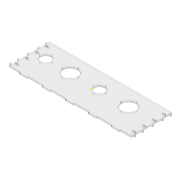
# Autodesk Inventor part: plano 1
Saved by Autodesk Inventor 2016 (Build 200138000, 138)
## iProperties
Created: 2017-08-31
Part Number: plano 1
Material: Vidrio
Document SubType Name: Modeling
Designer: Alumno
Density: 2.18 g/cm^3
Appearance: Claro
Author: Alumno
Autodesk Inventor part; units mm, degrees
ref_plane "YZ Plane" through (0, 0, 0) normal (1, 0, 0) x (0, 1, 0)
ref_plane "XZ Plane" through (0, 0, 0) normal (0, 1, 0) x (-1, 0, 0)
ref_plane "XY Plane" through (0, 0, 0) normal (0, 0, 1) x (1, 0, 0)
sketch "Boceto1" plane through (0, 0, 0) normal (0, 0, 1) x (1, 0, 0)
  line L0 (225, -75) -> (-225, -75)
  line L1 (-225, -75) -> (-225, 75)
  line L2 (-225, 75) -> (225, 75)
  line L3 (225, 75) -> (225, -75)
  line L4 (225, -75) -> (-225, 75) construction
  line L5 (-225, -75) -> (225, 75) construction
  point P0 (0, 0)
  dimension "d0" = 450
  dimension "d1" = 150
  constraints: 12 end point, 2 midpoint, 2 parallel, 1 horizontal, 1 perpendicular
  measures "d0" distance of L1.end L2.end
  measures "d1" distance of L0.end L1.end
extrude "Extrusión1" add sketch "Boceto1" along normal blind 6
sketch "Boceto2" plane through (0, 0, 6) normal (0, 0, 1) x (1, 0, 0)
  line L0 (-225, -75) -> (225, -75) projected
  line L1 (225, -75) -> (225, 75) projected
  line L2 (225, 75) -> (-225, 75) projected
  line L3 (-225, 75) -> (-225, -75) projected
  line L4 (-210, 57) -> (-210, 53.65)
  line L5 (-225, 53.65) -> (-225, 57)
  line L6 (-216, 52.35) -> (-218.8, 52.35)
  line L7 (-218.8, 58.3) -> (-216, 58.3)
  line L8 (-216, 58.3) -> (-216, 57)
  line L9 (-216, 53.65) -> (-216, 52.35)
  line L10 (-218.8, 52.35) -> (-218.8, 53.65)
  line L11 (-218.8, 57) -> (-218.8, 58.3)
  line L12 (-225, 57) -> (-218.8, 57)
  line L13 (-216, 57) -> (-210, 57)
  line L14 (-210, 53.65) -> (-216, 53.65)
  line L15 (-218.8, 53.65) -> (-225, 53.65)
  line L16 (-210, -53.65) -> (-210, -57)
  line L17 (-225, -57) -> (-225, -53.65)
  line L18 (-216, -58.3) -> (-218.8, -58.3)
  line L19 (-218.8, -52.35) -> (-216, -52.35)
  line L20 (-216, -52.35) -> (-216, -53.65)
  line L21 (-216, -57) -> (-216, -58.3)
  line L22 (-218.8, -58.3) -> (-218.8, -57)
  line L23 (-218.8, -53.65) -> (-218.8, -52.35)
  line L24 (-225, -53.65) -> (-218.8, -53.65)
  line L25 (-216, -53.65) -> (-210, -53.65)
  line L26 (-210, -57) -> (-216, -57)
  line L27 (-218.8, -57) -> (-225, -57)
  line L28 (-210, -16.7667) -> (-210, -20.1167)
  line L29 (-225, -20.1167) -> (-225, -16.7667)
  line L30 (-216, -15.4667) -> (-218.8, -15.4667)
  line L31 (-218.8, -21.4167) -> (-216, -21.4167)
  line L32 (-216, -16.7667) -> (-216, -15.4667)
  line L33 (-218.8, -15.4667) -> (-218.8, -16.7667)
  line L34 (-218.8, -20.1167) -> (-218.8, -21.4167)
  line L35 (-225, -16.7667) -> (-218.8, -16.7667)
  line L36 (-216, -16.7667) -> (-210, -16.7667)
  line L37 (-210, -20.1167) -> (-216, -20.1167)
  line L38 (-218.8, -20.1167) -> (-225, -20.1167)
  line L39 (-210, 20.1167) -> (-210, 16.7667)
  line L40 (-225, 16.7667) -> (-225, 20.1167)
  line L41 (-216, 15.4667) -> (-218.8, 15.4667)
  line L42 (-218.8, 21.4167) -> (-216, 21.4167)
  line L43 (-216, 21.4167) -> (-216, 20.1167)
  line L44 (-216, 16.7667) -> (-216, 15.4667)
  line L45 (-218.8, 15.4667) -> (-218.8, 16.7667)
  line L46 (-218.8, 20.1167) -> (-218.8, 21.4167)
  line L47 (-225, 20.1167) -> (-218.8, 20.1167)
  line L48 (-216, 20.1167) -> (-210, 20.1167)
  line L49 (-210, 16.7667) -> (-216, 16.7667)
  line L50 (-218.8, 16.7667) -> (-225, 16.7667)
  line L51 (-216, -21.4167) -> (-216, -20.1167)
  line L52 (-225, 75) -> (-225, -75) projected
  point P0 (0, 0)
  point P1 (-216.3708, 45.3131)
  point P2 (-225, 57)
  dimension "d5" = 3.35
  dimension "d6" = 2.8
  dimension "d8" = 6
  dimension "d9" = 6
  dimension "d11" = 3.35
  dimension "d12" = 18
  dimension "d46" = 15
  dimension "d47" = 3.35
  dimension "d48" = 2.8
  dimension "d49" = 2.8
  dimension "d52" = 3.35
  dimension "d53" = 15
  dimension "d54" = 3.35
  dimension "d60" = 15
  dimension "d61" = 3.35
  dimension "d62" = 2.8
  dimension "d63" = 2.8
  dimension "d66" = 3.35
  dimension "d67" = 18
  dimension "d71" = 107.3
  dimension "d72" = 33.5333
  dimension "d73" = 33.5333
  dimension "d74" = 5.95
  dimension "d76" = 5.95
  dimension "d77" = 1.3
  dimension "d78" = 5.95
  dimension "d79" = 1.3
  dimension "d80" = 1.3
  dimension "d81" = 1.3
  dimension "d137" = 3.35
  dimension "d138" = 6.2
  dimension "d139" = 2.8
  dimension "d140" = 15
  dimension "d141" = 6.2
  dimension "d142" = 6.2
  dimension "d143" = 6.2
  dimension "d144" = 6.2
  dimension "d145" = 2.8
  dimension "d146" = 2.8
  dimension "d147" = 6.2
  dimension "d148" = 6.2
  constraints: 96 end point, 38 parallel, 16 perpendicular, 12 horizontal, 1 coincident, 1 point on line, 1 vertical
  measures "d5" distance of L4.start L4.end
  measures "d6" distance of L6.start L6.end
  measures "d8" distance between parallel lines of L8 L4
  measures "d9" distance between parallel lines of L9 L4
  measures "d11" distance between parallel lines of L15 L12
  measures "d12" distance between parallel lines of L2 L12
  measures "d46" distance of L16.end L27.end
  measures "d47" distance of L16.start L16.end
  measures "d48" distance of L21.end L22.start
  measures "d49" distance of L23.end L20.start
  measures "d52" distance between parallel lines of L27 L24
  measures "d53" distance of L28.end L38.end
  measures "d54" distance of L28.start L28.end
  measures "d60" distance of L39.end L50.end
  measures "d61" distance of L39.start L39.end
  measures "d62" distance of L44.end L45.start
  measures "d63" distance of L46.end L43.start
  measures "d66" distance between parallel lines of L50 L47
  measures "d67" distance between parallel lines of L0 L27
  measures "d71" distance between parallel lines of L24 L15
  measures "d72" distance between parallel lines of L47 L15
  measures "d73" distance between parallel lines of L35 L50
  measures "d74" distance between parallel lines of L18 L19
  measures "d76" distance between parallel lines of L6 L7
  measures "d77" distance between parallel lines of L48 L42
  measures "d78" distance between parallel lines of L41 L42
  measures "d79" distance between parallel lines of L35 L30
  measures "d80" distance between parallel lines of L31 L38
  measures "d81" distance between parallel lines of L24 L19
  measures "d137" distance between parallel lines of L14 L13
  measures "d138" distance of L5.end L11.start
  measures "d139" distance of L7.start L7.end
  measures "d140" distance between parallel lines of L4 L52
  measures "d141" distance of L47.start L46.start
  measures "d142" distance of L45.end L50.end
  measures "d143" distance of L35.start L33.end
  measures "d144" distance of L34.start L38.end
  measures "d145" distance of L32.end L33.start
  measures "d146" distance of L34.end L31.end
  measures "d147" distance of L24.start L23.start
  measures "d148" distance of L22.end L27.end
extrude "Extrusión2" cut sketch "Boceto2" against normal blind 6 contours L3 L24 L23 L19 L20 L25 L16 L26 L21 L18 L22 L27 | L12 L11 L7 L8 L13 L4 L14 L9 L6 L10 L15 L3 | L3 L47 L46 L42 L43 L48 L39 L49 L44 L41 L45 L50
extrude "Extrusión3" cut sketch "Boceto2" against normal blind 6 contours L3 L35 L33 L30 L32 L36 L28 L37 L51 L31 L34 L38
mirror "Simetría1" about plane through (0, 0, 0) normal (1, 0, 0) of "Extrusión3", "Extrusión2"
sketch "Boceto3" plane through (0, 0, 6) normal (0, 0, 1) x (1, 0, 0)
  line L0 (-225, -75) -> (225, -75) projected
  line L1 (-225, 75) -> (-225, -75) projected
  circle A0 centre (-180, 15) radius 19
  circle A1 centre (-90, 15) radius 21.5
  circle A2 centre (18, 15) radius 19
  circle A3 centre (126, 15) radius 21.5
  point P0 (-225, 53.65)
  point P1 (-225, 20.1167)
  dimension "d97" = 90
  dimension "d98" = 45
  dimension "d99" = 90
  dimension "d100" = 108
  dimension "d101" = 108
  dimension "d102" = 38
  dimension "d105" = 43
  dimension "d108" = 38
  dimension "d109" = 43
  constraints: 4 centre point, 4 coincident
  measures "d97" distance from line of L0 point (-180, 15)
  measures "d98" distance from line of L1 point (-180, 15)
  measures "d99" distance of point (-90, 15) point (-180, 15)
  measures "d100" distance of point (18, 15) point (-90, 15)
  measures "d101" distance of point (126, 15) point (18, 15)
  measures "d102" diameter of A0
  measures "d105" diameter of A1
  measures "d108" diameter of A2
  measures "d109" diameter of A3
extrude "Extrusión4" cut sketch "Boceto3" against normal blind 10 contours A0
extrude "Extrusión5" cut sketch "Boceto3" against normal blind 10 contours A1
extrude "Extrusión6" cut sketch "Boceto3" against normal blind 10 contours A2 | A3
sketch "Boceto4" plane through (0, 0, 6) normal (0, 0, 1) x (1, 0, 0)
  circle A0 centre (18, 15) radius 19 projected
  circle A1 centre (126, 15) radius 21.5 projected
  circle A2 centre (-90, 15) radius 21.5 projected
  circle A3 centre (-180, 15) radius 19 projected
  line L0 (225, 16.7667) -> (218.8, 16.7667) projected
  line L1 (218.8, 16.7667) -> (218.8, 15.4667) projected
  line L2 (218.8, 15.4667) -> (216, 15.4667) projected
  line L3 (216, 15.4667) -> (216, 16.7667) projected
  line L4 (216, 16.7667) -> (210, 16.7667) projected
  line L5 (210, 16.7667) -> (210, 20.1167) projected
  line L6 (210, 20.1167) -> (216, 20.1167) projected
  line L7 (216, 20.1167) -> (216, 21.4167) projected
  line L8 (216, 21.4167) -> (218.8, 21.4167) projected
  line L9 (218.8, 21.4167) -> (218.8, 20.1167) projected
  line L10 (218.8, 20.1167) -> (225, 20.1167) projected
  line L11 (225, 20.1167) -> (225, 53.65) projected
  line L12 (225, 53.65) -> (218.8, 53.65) projected
  line L13 (218.8, 53.65) -> (218.8, 52.35) projected
  line L14 (218.8, 52.35) -> (216, 52.35) projected
  line L15 (216, 52.35) -> (216, 53.65) projected
  line L16 (216, 53.65) -> (210, 53.65) projected
  line L17 (210, 53.65) -> (210, 57) projected
  line L18 (210, 57) -> (216, 57) projected
  line L19 (216, 57) -> (216, 58.3) projected
  line L20 (216, 58.3) -> (218.8, 58.3) projected
  line L21 (218.8, 58.3) -> (218.8, 57) projected
  line L22 (218.8, 57) -> (225, 57) projected
  line L23 (225, 57) -> (225, 75) projected
  line L24 (225, 75) -> (-225, 75) projected
  line L25 (-225, 75) -> (-225, 57) projected
  line L26 (-225, 57) -> (-218.8, 57) projected
  line L27 (-218.8, 57) -> (-218.8, 58.3) projected
  line L28 (-218.8, 58.3) -> (-216, 58.3) projected
  line L29 (-216, 58.3) -> (-216, 57) projected
  line L30 (-216, 57) -> (-210, 57) projected
  line L31 (-210, 57) -> (-210, 53.65) projected
  line L32 (-210, 53.65) -> (-216, 53.65) projected
  line L33 (-216, 53.65) -> (-216, 52.35) projected
  line L34 (-216, 52.35) -> (-218.8, 52.35) projected
  line L35 (-218.8, 52.35) -> (-218.8, 53.65) projected
  line L36 (-218.8, 53.65) -> (-225, 53.65) projected
  line L37 (-225, 53.65) -> (-225, 20.1167) projected
  line L38 (-225, 20.1167) -> (-218.8, 20.1167) projected
  line L39 (-218.8, 20.1167) -> (-218.8, 21.4167) projected
  line L40 (-218.8, 21.4167) -> (-216, 21.4167) projected
  line L41 (-216, 21.4167) -> (-216, 20.1167) projected
  line L42 (-216, 20.1167) -> (-210, 20.1167) projected
  line L43 (-210, 20.1167) -> (-210, 16.7667) projected
  line L44 (-210, 16.7667) -> (-216, 16.7667) projected
  line L45 (-216, 16.7667) -> (-216, 15.4667) projected
  line L46 (-216, 15.4667) -> (-218.8, 15.4667) projected
  line L47 (-218.8, 15.4667) -> (-218.8, 16.7667) projected
  line L48 (-218.8, 16.7667) -> (-225, 16.7667) projected
  line L49 (-225, 16.7667) -> (-225, -16.7667) projected
  line L50 (-225, -16.7667) -> (-218.8, -16.7667) projected
  line L51 (-218.8, -16.7667) -> (-218.8, -15.4667) projected
  line L52 (-218.8, -15.4667) -> (-216, -15.4667) projected
  line L53 (-216, -15.4667) -> (-216, -16.7667) projected
  line L54 (-216, -16.7667) -> (-210, -16.7667) projected
  line L55 (-210, -16.7667) -> (-210, -20.1167) projected
  line L56 (-210, -20.1167) -> (-216, -20.1167) projected
  line L57 (-216, -20.1167) -> (-216, -21.4167) projected
  line L58 (-216, -21.4167) -> (-218.8, -21.4167) projected
  line L59 (-218.8, -21.4167) -> (-218.8, -20.1167) projected
  line L60 (-218.8, -20.1167) -> (-225, -20.1167) projected
  line L61 (-225, -20.1167) -> (-225, -53.65) projected
  line L62 (-225, -53.65) -> (-218.8, -53.65) projected
  line L63 (-218.8, -53.65) -> (-218.8, -52.35) projected
  line L64 (-218.8, -52.35) -> (-216, -52.35) projected
  line L65 (-216, -52.35) -> (-216, -53.65) projected
  line L66 (-216, -53.65) -> (-210, -53.65) projected
  line L67 (-210, -53.65) -> (-210, -57) projected
  line L68 (-210, -57) -> (-216, -57) projected
  line L69 (-216, -57) -> (-216, -58.3) projected
  line L70 (-216, -58.3) -> (-218.8, -58.3) projected
  line L71 (-218.8, -58.3) -> (-218.8, -57) projected
  line L72 (-218.8, -57) -> (-225, -57) projected
  line L73 (-225, -57) -> (-225, -75) projected
  line L74 (-225, -75) -> (225, -75) projected
  line L75 (225, -75) -> (225, -57) projected
  line L76 (225, -57) -> (218.8, -57) projected
  line L77 (218.8, -57) -> (218.8, -58.3) projected
  line L78 (218.8, -58.3) -> (216, -58.3) projected
  line L79 (216, -58.3) -> (216, -57) projected
  line L80 (216, -57) -> (210, -57) projected
  line L81 (210, -57) -> (210, -53.65) projected
  line L82 (210, -53.65) -> (216, -53.65) projected
  line L83 (216, -53.65) -> (216, -52.35) projected
  line L84 (216, -52.35) -> (218.8, -52.35) projected
  line L85 (218.8, -52.35) -> (218.8, -53.65) projected
  line L86 (218.8, -53.65) -> (225, -53.65) projected
  line L87 (225, -53.65) -> (225, -20.1167) projected
  line L88 (225, -20.1167) -> (218.8, -20.1167) projected
  line L89 (218.8, -20.1167) -> (218.8, -21.4167) projected
  line L90 (218.8, -21.4167) -> (216, -21.4167) projected
  line L91 (216, -21.4167) -> (216, -20.1167) projected
  line L92 (216, -20.1167) -> (210, -20.1167) projected
  line L93 (210, -20.1167) -> (210, -16.7667) projected
  line L94 (210, -16.7667) -> (216, -16.7667) projected
  line L95 (216, -16.7667) -> (216, -15.4667) projected
  line L96 (216, -15.4667) -> (218.8, -15.4667) projected
  line L97 (218.8, -15.4667) -> (218.8, -16.7667) projected
  line L98 (218.8, -16.7667) -> (225, -16.7667) projected
  line L99 (225, -16.7667) -> (225, 16.7667) projected
  line L100 (-225, 57) -> (-225, 75) projected
  line L101 (-225, 63.9297) -> (-225, 68.9297)
  line L102 (-225, 53.65) -> (-225, 20.1167) projected
  line L103 (-230, 2.5) -> (-225, 2.5)
  line L104 (-225, 2.5) -> (-225, -2.5)
  line L105 (-225, -2.5) -> (-230, -2.5)
  line L106 (-230, -2.5) -> (-230, 2.5)
  line L107 (-230, -34.3833) -> (-225, -34.3833)
  line L108 (-225, -34.3833) -> (-225, -39.3833)
  line L109 (-225, -39.3833) -> (-230, -39.3833)
  line L110 (-230, -39.3833) -> (-230, -34.3833)
  line L111 (-230, -63.5) -> (-225, -63.5)
  line L112 (-225, -63.5) -> (-225, -68.5)
  line L113 (-225, -68.5) -> (-230, -68.5)
  line L114 (-230, -68.5) -> (-230, -63.5)
  line L115 (-230, 68.9297) -> (-225, 68.9297)
  line L116 (-225, 68.9297) -> (-225, 63.9297)
  line L117 (-225, 63.9297) -> (-230, 63.9297)
  line L118 (-230, 63.9297) -> (-230, 68.9297)
  line L119 (-230, 39.3833) -> (-225, 39.3833)
  line L120 (-225, 39.3833) -> (-225, 34.3833)
  line L121 (-225, 34.3833) -> (-230, 34.3833)
  line L122 (-230, 34.3833) -> (-230, 39.3833)
  point P0 (0, 0)
  point P1 (-225, 0)
  point P2 (-225, -36.8833)
  point P3 (-225, -66)
  point P4 (-225, 66.4297)
  point P5 (-225, 36.8833)
  dimension "d116" = 5
  dimension "d117" = 5
  dimension "d118" = 5
  dimension "d119" = 5
  dimension "d120" = 5
  dimension "d121" = 5
  dimension "d122" = 5
  dimension "d123" = 5
  dimension "d124" = 5
  dimension "d125" = 5
  constraints: 42 end point, 10 midpoint, 10 parallel, 5 horizontal, 5 perpendicular, 1 point on line
  measures "d116" distance of L104.end L105.end
  measures "d117" distance of L103.end L104.end
  measures "d118" distance of L108.end L109.end
  measures "d119" distance of L107.end L108.end
  measures "d120" distance of L112.end L113.end
  measures "d121" distance of L111.end L112.end
  measures "d122" distance of L116.end L117.end
  measures "d123" distance of L115.end L116.end
  measures "d124" distance of L120.end L121.end
  measures "d125" distance of L119.end L120.end
extrude "Extrusión7" add sketch "Boceto4" against normal blind 6 contours L25 L117 L118 L115 | L113 L114 L111 L73 | L37 L121 L122 L119 | L109 L110 L107 L61 | L49 L105 L106 L103
mirror "Simetría2" about plane through (0, 0, 0) normal (1, 0, 0) of "Extrusión7"
sketch "Boceto6" plane through (0, 0, 6) normal (0, 0, 1) x (1, 0, 0)
  circle A0 centre (18, 15) radius 19 projected
  circle A1 centre (126, 15) radius 21.5 projected
  circle A2 centre (-90, 15) radius 21.5 projected
  circle A3 centre (-180, 15) radius 19 projected
  line L0 (225, 16.7667) -> (218.8, 16.7667) projected
  line L1 (218.8, 16.7667) -> (218.8, 15.4667) projected
  line L2 (218.8, 15.4667) -> (216, 15.4667) projected
  line L3 (216, 15.4667) -> (216, 16.7667) projected
  line L4 (216, 16.7667) -> (210, 16.7667) projected
  line L5 (210, 16.7667) -> (210, 20.1167) projected
  line L6 (210, 20.1167) -> (216, 20.1167) projected
  line L7 (216, 20.1167) -> (216, 21.4167) projected
  line L8 (216, 21.4167) -> (218.8, 21.4167) projected
  line L9 (218.8, 21.4167) -> (218.8, 20.1167) projected
  line L10 (218.8, 20.1167) -> (225, 20.1167) projected
  line L11 (225, 20.1167) -> (225, 34.3833) projected
  line L12 (230, 34.3833) -> (225, 34.3833) projected
  line L13 (230, 39.3833) -> (230, 34.3833) projected
  line L14 (225, 39.3833) -> (230, 39.3833) projected
  line L15 (225, 39.3833) -> (225, 53.65) projected
  line L16 (225, 53.65) -> (218.8, 53.65) projected
  line L17 (218.8, 53.65) -> (218.8, 52.35) projected
  line L18 (218.8, 52.35) -> (216, 52.35) projected
  line L19 (216, 52.35) -> (216, 53.65) projected
  line L20 (216, 53.65) -> (210, 53.65) projected
  line L21 (210, 53.65) -> (210, 57) projected
  line L22 (210, 57) -> (216, 57) projected
  line L23 (216, 57) -> (216, 58.3) projected
  line L24 (216, 58.3) -> (218.8, 58.3) projected
  line L25 (218.8, 58.3) -> (218.8, 57) projected
  line L26 (218.8, 57) -> (225, 57) projected
  line L27 (225, 57) -> (225, 63.9297) projected
  line L28 (230, 63.9297) -> (225, 63.9297) projected
  line L29 (230, 68.9297) -> (230, 63.9297) projected
  line L30 (225, 68.9297) -> (230, 68.9297) projected
  line L31 (225, 68.9297) -> (225, 75) projected
  line L32 (225, 75) -> (-225, 75) projected
  line L33 (-225, 75) -> (-225, 68.9297) projected
  line L34 (-225, 68.9297) -> (-230, 68.9297) projected
  line L35 (-230, 68.9297) -> (-230, 63.9297) projected
  line L36 (-230, 63.9297) -> (-225, 63.9297) projected
  line L37 (-225, 63.9297) -> (-225, 57) projected
  line L38 (-225, 57) -> (-218.8, 57) projected
  line L39 (-218.8, 57) -> (-218.8, 58.3) projected
  line L40 (-218.8, 58.3) -> (-216, 58.3) projected
  line L41 (-216, 58.3) -> (-216, 57) projected
  line L42 (-216, 57) -> (-210, 57) projected
  line L43 (-210, 57) -> (-210, 53.65) projected
  line L44 (-210, 53.65) -> (-216, 53.65) projected
  line L45 (-216, 53.65) -> (-216, 52.35) projected
  line L46 (-216, 52.35) -> (-218.8, 52.35) projected
  line L47 (-218.8, 52.35) -> (-218.8, 53.65) projected
  line L48 (-218.8, 53.65) -> (-225, 53.65) projected
  line L49 (-225, 53.65) -> (-225, 39.3833) projected
  line L50 (-225, 39.3833) -> (-230, 39.3833) projected
  line L51 (-230, 39.3833) -> (-230, 34.3833) projected
  line L52 (-230, 34.3833) -> (-225, 34.3833) projected
  line L53 (-225, 34.3833) -> (-225, 20.1167) projected
  line L54 (-225, 20.1167) -> (-218.8, 20.1167) projected
  line L55 (-218.8, 20.1167) -> (-218.8, 21.4167) projected
  line L56 (-218.8, 21.4167) -> (-216, 21.4167) projected
  line L57 (-216, 21.4167) -> (-216, 20.1167) projected
  line L58 (-216, 20.1167) -> (-210, 20.1167) projected
  line L59 (-210, 20.1167) -> (-210, 16.7667) projected
  line L60 (-210, 16.7667) -> (-216, 16.7667) projected
  line L61 (-216, 16.7667) -> (-216, 15.4667) projected
  line L62 (-216, 15.4667) -> (-218.8, 15.4667) projected
  line L63 (-218.8, 15.4667) -> (-218.8, 16.7667) projected
  line L64 (-218.8, 16.7667) -> (-225, 16.7667) projected
  line L65 (-225, 16.7667) -> (-225, 2.5) projected
  line L66 (-225, 2.5) -> (-230, 2.5) projected
  line L67 (-230, 2.5) -> (-230, -2.5) projected
  line L68 (-230, -2.5) -> (-225, -2.5) projected
  line L69 (-225, -2.5) -> (-225, -16.7667) projected
  line L70 (-225, -16.7667) -> (-218.8, -16.7667) projected
  line L71 (-218.8, -16.7667) -> (-218.8, -15.4667) projected
  line L72 (-218.8, -15.4667) -> (-216, -15.4667) projected
  line L73 (-216, -15.4667) -> (-216, -16.7667) projected
  line L74 (-216, -16.7667) -> (-210, -16.7667) projected
  line L75 (-210, -16.7667) -> (-210, -20.1167) projected
  line L76 (-210, -20.1167) -> (-216, -20.1167) projected
  line L77 (-216, -20.1167) -> (-216, -21.4167) projected
  line L78 (-216, -21.4167) -> (-218.8, -21.4167) projected
  line L79 (-218.8, -21.4167) -> (-218.8, -20.1167) projected
  line L80 (-218.8, -20.1167) -> (-225, -20.1167) projected
  line L81 (-225, -20.1167) -> (-225, -34.3833) projected
  line L82 (-225, -34.3833) -> (-230, -34.3833) projected
  line L83 (-230, -34.3833) -> (-230, -39.3833) projected
  line L84 (-230, -39.3833) -> (-225, -39.3833) projected
  line L85 (-225, -39.3833) -> (-225, -53.65) projected
  line L86 (-225, -53.65) -> (-218.8, -53.65) projected
  line L87 (-218.8, -53.65) -> (-218.8, -52.35) projected
  line L88 (-218.8, -52.35) -> (-216, -52.35) projected
  line L89 (-216, -52.35) -> (-216, -53.65) projected
  line L90 (-216, -53.65) -> (-210, -53.65) projected
  line L91 (-210, -53.65) -> (-210, -57) projected
  line L92 (-210, -57) -> (-216, -57) projected
  line L93 (-216, -57) -> (-216, -58.3) projected
  line L94 (-216, -58.3) -> (-218.8, -58.3) projected
  line L95 (-218.8, -58.3) -> (-218.8, -57) projected
  line L96 (-218.8, -57) -> (-225, -57) projected
  line L97 (-225, -57) -> (-225, -63.5) projected
  line L98 (-225, -63.5) -> (-230, -63.5) projected
  line L99 (-230, -63.5) -> (-230, -68.5) projected
  line L100 (-230, -68.5) -> (-225, -68.5) projected
  line L101 (-225, -68.5) -> (-225, -75) projected
  line L102 (-225, -75) -> (225, -75) projected
  line L103 (225, -75) -> (225, -68.5) projected
  line L104 (230, -68.5) -> (225, -68.5) projected
  line L105 (230, -63.5) -> (230, -68.5) projected
  line L106 (225, -63.5) -> (230, -63.5) projected
  line L107 (225, -63.5) -> (225, -57) projected
  line L108 (225, -57) -> (218.8, -57) projected
  line L109 (218.8, -57) -> (218.8, -58.3) projected
  line L110 (218.8, -58.3) -> (216, -58.3) projected
  line L111 (216, -58.3) -> (216, -57) projected
  line L112 (216, -57) -> (210, -57) projected
  line L113 (210, -57) -> (210, -53.65) projected
  line L114 (210, -53.65) -> (216, -53.65) projected
  line L115 (216, -53.65) -> (216, -52.35) projected
  line L116 (216, -52.35) -> (218.8, -52.35) projected
  line L117 (218.8, -52.35) -> (218.8, -53.65) projected
  line L118 (218.8, -53.65) -> (225, -53.65) projected
  line L119 (225, -53.65) -> (225, -39.3833) projected
  line L120 (230, -39.3833) -> (225, -39.3833) projected
  line L121 (230, -34.3833) -> (230, -39.3833) projected
  line L122 (225, -34.3833) -> (230, -34.3833) projected
  line L123 (225, -34.3833) -> (225, -20.1167) projected
  line L124 (225, -20.1167) -> (218.8, -20.1167) projected
  line L125 (218.8, -20.1167) -> (218.8, -21.4167) projected
  line L126 (218.8, -21.4167) -> (216, -21.4167) projected
  line L127 (216, -21.4167) -> (216, -20.1167) projected
  line L128 (216, -20.1167) -> (210, -20.1167) projected
  line L129 (210, -20.1167) -> (210, -16.7667) projected
  line L130 (210, -16.7667) -> (216, -16.7667) projected
  line L131 (216, -16.7667) -> (216, -15.4667) projected
  line L132 (216, -15.4667) -> (218.8, -15.4667) projected
  line L133 (218.8, -15.4667) -> (218.8, -16.7667) projected
  line L134 (218.8, -16.7667) -> (225, -16.7667) projected
  line L135 (225, -16.7667) -> (225, -2.5) projected
  line L136 (230, -2.5) -> (225, -2.5) projected
  line L137 (230, 2.5) -> (230, -2.5) projected
  line L138 (225, 2.5) -> (230, 2.5) projected
  line L139 (225, 2.5) -> (225, 16.7667) projected
  circle A4 centre (-180, 15) radius 14
  circle A5 centre (-180, 15) radius 25
  circle A6 centre (18, 38) radius 1.5
  circle A7 centre (18, 15) radius 14
  circle A8 centre (18, 15) radius 25
  circle A9 centre (-5, 15) radius 1.5
  circle A10 centre (18, -8) radius 1.5
  circle A11 centre (41, 15) radius 1.5
  circle A12 centre (-180, 38) radius 1.5
  circle A13 centre (-203, 15) radius 1.5
  circle A14 centre (-180, -8) radius 1.5
  circle A15 centre (-157, 15) radius 1.5
  point P0 (0, 0)
  dimension "d149" = 23
  dimension "d152" = 360
  dimension "d157" = 3
  dimension "d158" = 23
  dimension "d161" = 360
  constraints: 12 centre point, 18 other
  measures "d149" distance of A0.centre A6.centre
  measures "d157" diameter of A12
  measures "d158" distance of A3.centre A12.centre
sketch "Boceto7" plane through (0, 0, 6) normal (0, 0, 1) x (1, 0, 0)
  circle A0 centre (18, 15) radius 19 projected
  circle A1 centre (126, 15) radius 21.5 projected
  circle A2 centre (-90, 15) radius 21.5 projected
  circle A3 centre (-180, 15) radius 19 projected
  line L0 (225, 16.7667) -> (218.8, 16.7667) projected
  line L1 (218.8, 16.7667) -> (218.8, 15.4667) projected
  line L2 (218.8, 15.4667) -> (216, 15.4667) projected
  line L3 (216, 15.4667) -> (216, 16.7667) projected
  line L4 (216, 16.7667) -> (210, 16.7667) projected
  line L5 (210, 16.7667) -> (210, 20.1167) projected
  line L6 (210, 20.1167) -> (216, 20.1167) projected
  line L7 (216, 20.1167) -> (216, 21.4167) projected
  line L8 (216, 21.4167) -> (218.8, 21.4167) projected
  line L9 (218.8, 21.4167) -> (218.8, 20.1167) projected
  line L10 (218.8, 20.1167) -> (225, 20.1167) projected
  line L11 (225, 20.1167) -> (225, 34.3833) projected
  line L12 (230, 34.3833) -> (225, 34.3833) projected
  line L13 (230, 39.3833) -> (230, 34.3833) projected
  line L14 (225, 39.3833) -> (230, 39.3833) projected
  line L15 (225, 39.3833) -> (225, 53.65) projected
  line L16 (225, 53.65) -> (218.8, 53.65) projected
  line L17 (218.8, 53.65) -> (218.8, 52.35) projected
  line L18 (218.8, 52.35) -> (216, 52.35) projected
  line L19 (216, 52.35) -> (216, 53.65) projected
  line L20 (216, 53.65) -> (210, 53.65) projected
  line L21 (210, 53.65) -> (210, 57) projected
  line L22 (210, 57) -> (216, 57) projected
  line L23 (216, 57) -> (216, 58.3) projected
  line L24 (216, 58.3) -> (218.8, 58.3) projected
  line L25 (218.8, 58.3) -> (218.8, 57) projected
  line L26 (218.8, 57) -> (225, 57) projected
  line L27 (225, 57) -> (225, 63.9297) projected
  line L28 (230, 63.9297) -> (225, 63.9297) projected
  line L29 (230, 68.9297) -> (230, 63.9297) projected
  line L30 (225, 68.9297) -> (230, 68.9297) projected
  line L31 (225, 68.9297) -> (225, 75) projected
  line L32 (225, 75) -> (-225, 75) projected
  line L33 (-225, 75) -> (-225, 68.9297) projected
  line L34 (-225, 68.9297) -> (-230, 68.9297) projected
  line L35 (-230, 68.9297) -> (-230, 63.9297) projected
  line L36 (-230, 63.9297) -> (-225, 63.9297) projected
  line L37 (-225, 63.9297) -> (-225, 57) projected
  line L38 (-225, 57) -> (-218.8, 57) projected
  line L39 (-218.8, 57) -> (-218.8, 58.3) projected
  line L40 (-218.8, 58.3) -> (-216, 58.3) projected
  line L41 (-216, 58.3) -> (-216, 57) projected
  line L42 (-216, 57) -> (-210, 57) projected
  line L43 (-210, 57) -> (-210, 53.65) projected
  line L44 (-210, 53.65) -> (-216, 53.65) projected
  line L45 (-216, 53.65) -> (-216, 52.35) projected
  line L46 (-216, 52.35) -> (-218.8, 52.35) projected
  line L47 (-218.8, 52.35) -> (-218.8, 53.65) projected
  line L48 (-218.8, 53.65) -> (-225, 53.65) projected
  line L49 (-225, 53.65) -> (-225, 39.3833) projected
  line L50 (-225, 39.3833) -> (-230, 39.3833) projected
  line L51 (-230, 39.3833) -> (-230, 34.3833) projected
  line L52 (-230, 34.3833) -> (-225, 34.3833) projected
  line L53 (-225, 34.3833) -> (-225, 20.1167) projected
  line L54 (-225, 20.1167) -> (-218.8, 20.1167) projected
  line L55 (-218.8, 20.1167) -> (-218.8, 21.4167) projected
  line L56 (-218.8, 21.4167) -> (-216, 21.4167) projected
  line L57 (-216, 21.4167) -> (-216, 20.1167) projected
  line L58 (-216, 20.1167) -> (-210, 20.1167) projected
  line L59 (-210, 20.1167) -> (-210, 16.7667) projected
  line L60 (-210, 16.7667) -> (-216, 16.7667) projected
  line L61 (-216, 16.7667) -> (-216, 15.4667) projected
  line L62 (-216, 15.4667) -> (-218.8, 15.4667) projected
  line L63 (-218.8, 15.4667) -> (-218.8, 16.7667) projected
  line L64 (-218.8, 16.7667) -> (-225, 16.7667) projected
  line L65 (-225, 16.7667) -> (-225, 2.5) projected
  line L66 (-225, 2.5) -> (-230, 2.5) projected
  line L67 (-230, 2.5) -> (-230, -2.5) projected
  line L68 (-230, -2.5) -> (-225, -2.5) projected
  line L69 (-225, -2.5) -> (-225, -16.7667) projected
  line L70 (-225, -16.7667) -> (-218.8, -16.7667) projected
  line L71 (-218.8, -16.7667) -> (-218.8, -15.4667) projected
  line L72 (-218.8, -15.4667) -> (-216, -15.4667) projected
  line L73 (-216, -15.4667) -> (-216, -16.7667) projected
  line L74 (-216, -16.7667) -> (-210, -16.7667) projected
  line L75 (-210, -16.7667) -> (-210, -20.1167) projected
  line L76 (-210, -20.1167) -> (-216, -20.1167) projected
  line L77 (-216, -20.1167) -> (-216, -21.4167) projected
  line L78 (-216, -21.4167) -> (-218.8, -21.4167) projected
  line L79 (-218.8, -21.4167) -> (-218.8, -20.1167) projected
  line L80 (-218.8, -20.1167) -> (-225, -20.1167) projected
  line L81 (-225, -20.1167) -> (-225, -34.3833) projected
  line L82 (-225, -34.3833) -> (-230, -34.3833) projected
  line L83 (-230, -34.3833) -> (-230, -39.3833) projected
  line L84 (-230, -39.3833) -> (-225, -39.3833) projected
  line L85 (-225, -39.3833) -> (-225, -53.65) projected
  line L86 (-225, -53.65) -> (-218.8, -53.65) projected
  line L87 (-218.8, -53.65) -> (-218.8, -52.35) projected
  line L88 (-218.8, -52.35) -> (-216, -52.35) projected
  line L89 (-216, -52.35) -> (-216, -53.65) projected
  line L90 (-216, -53.65) -> (-210, -53.65) projected
  line L91 (-210, -53.65) -> (-210, -57) projected
  line L92 (-210, -57) -> (-216, -57) projected
  line L93 (-216, -57) -> (-216, -58.3) projected
  line L94 (-216, -58.3) -> (-218.8, -58.3) projected
  line L95 (-218.8, -58.3) -> (-218.8, -57) projected
  line L96 (-218.8, -57) -> (-225, -57) projected
  line L97 (-225, -57) -> (-225, -63.5) projected
  line L98 (-225, -63.5) -> (-230, -63.5) projected
  line L99 (-230, -63.5) -> (-230, -68.5) projected
  line L100 (-230, -68.5) -> (-225, -68.5) projected
  line L101 (-225, -68.5) -> (-225, -75) projected
  line L102 (-225, -75) -> (225, -75) projected
  line L103 (225, -75) -> (225, -68.5) projected
  line L104 (230, -68.5) -> (225, -68.5) projected
  line L105 (230, -63.5) -> (230, -68.5) projected
  line L106 (225, -63.5) -> (230, -63.5) projected
  line L107 (225, -63.5) -> (225, -57) projected
  line L108 (225, -57) -> (218.8, -57) projected
  line L109 (218.8, -57) -> (218.8, -58.3) projected
  line L110 (218.8, -58.3) -> (216, -58.3) projected
  line L111 (216, -58.3) -> (216, -57) projected
  line L112 (216, -57) -> (210, -57) projected
  line L113 (210, -57) -> (210, -53.65) projected
  line L114 (210, -53.65) -> (216, -53.65) projected
  line L115 (216, -53.65) -> (216, -52.35) projected
  line L116 (216, -52.35) -> (218.8, -52.35) projected
  line L117 (218.8, -52.35) -> (218.8, -53.65) projected
  line L118 (218.8, -53.65) -> (225, -53.65) projected
  line L119 (225, -53.65) -> (225, -39.3833) projected
  line L120 (230, -39.3833) -> (225, -39.3833) projected
  line L121 (230, -34.3833) -> (230, -39.3833) projected
  line L122 (225, -34.3833) -> (230, -34.3833) projected
  line L123 (225, -34.3833) -> (225, -20.1167) projected
  line L124 (225, -20.1167) -> (218.8, -20.1167) projected
  line L125 (218.8, -20.1167) -> (218.8, -21.4167) projected
  line L126 (218.8, -21.4167) -> (216, -21.4167) projected
  line L127 (216, -21.4167) -> (216, -20.1167) projected
  line L128 (216, -20.1167) -> (210, -20.1167) projected
  line L129 (210, -20.1167) -> (210, -16.7667) projected
  line L130 (210, -16.7667) -> (216, -16.7667) projected
  line L131 (216, -16.7667) -> (216, -15.4667) projected
  line L132 (216, -15.4667) -> (218.8, -15.4667) projected
  line L133 (218.8, -15.4667) -> (218.8, -16.7667) projected
  line L134 (218.8, -16.7667) -> (225, -16.7667) projected
  line L135 (225, -16.7667) -> (225, -2.5) projected
  line L136 (230, -2.5) -> (225, -2.5) projected
  line L137 (230, 2.5) -> (230, -2.5) projected
  line L138 (225, 2.5) -> (230, 2.5) projected
  line L139 (225, 2.5) -> (225, 16.7667) projected
  circle A4 centre (-90, 45) radius 1.5
  circle A5 centre (-90, 15) radius 18.5
  circle A6 centre (126, 45) radius 1.5
  circle A7 centre (126, 15) radius 18.5
  circle A8 centre (-120, 15) radius 1.5
  circle A9 centre (-90, -15) radius 1.5
  circle A10 centre (-60, 15) radius 1.5
  circle A11 centre (96, 15) radius 1.5
  circle A12 centre (126, -15) radius 1.5
  circle A13 centre (156, 15) radius 1.5
  dimension "d165" = 30
  dimension "d168" = 360
  dimension "d170" = 30
  dimension "d173" = 360
  constraints: 10 centre point, 18 other
  measures "d165" distance of A2.centre A4.centre
  measures "d170" distance of A1.centre A6.centre
sketch "Boceto9" plane through (0, 0, 6) normal (0, 0, 1) x (1, 0, 0)
  circle A0 centre (18, 15) radius 19 projected
  circle A1 centre (126, 15) radius 21.5 projected
  circle A2 centre (-90, 15) radius 21.5 projected
  circle A3 centre (-180, 15) radius 19 projected
  line L0 (225, 16.7667) -> (218.8, 16.7667) projected
  line L1 (218.8, 16.7667) -> (218.8, 15.4667) projected
  line L2 (218.8, 15.4667) -> (216, 15.4667) projected
  line L3 (216, 15.4667) -> (216, 16.7667) projected
  line L4 (216, 16.7667) -> (210, 16.7667) projected
  line L5 (210, 16.7667) -> (210, 20.1167) projected
  line L6 (210, 20.1167) -> (216, 20.1167) projected
  line L7 (216, 20.1167) -> (216, 21.4167) projected
  line L8 (216, 21.4167) -> (218.8, 21.4167) projected
  line L9 (218.8, 21.4167) -> (218.8, 20.1167) projected
  line L10 (218.8, 20.1167) -> (225, 20.1167) projected
  line L11 (225, 20.1167) -> (225, 34.3833) projected
  line L12 (230, 34.3833) -> (225, 34.3833) projected
  line L13 (230, 39.3833) -> (230, 34.3833) projected
  line L14 (225, 39.3833) -> (230, 39.3833) projected
  line L15 (225, 39.3833) -> (225, 53.65) projected
  line L16 (225, 53.65) -> (218.8, 53.65) projected
  line L17 (218.8, 53.65) -> (218.8, 52.35) projected
  line L18 (218.8, 52.35) -> (216, 52.35) projected
  line L19 (216, 52.35) -> (216, 53.65) projected
  line L20 (216, 53.65) -> (210, 53.65) projected
  line L21 (210, 53.65) -> (210, 57) projected
  line L22 (210, 57) -> (216, 57) projected
  line L23 (216, 57) -> (216, 58.3) projected
  line L24 (216, 58.3) -> (218.8, 58.3) projected
  line L25 (218.8, 58.3) -> (218.8, 57) projected
  line L26 (218.8, 57) -> (225, 57) projected
  line L27 (225, 57) -> (225, 63.9297) projected
  line L28 (230, 63.9297) -> (225, 63.9297) projected
  line L29 (230, 68.9297) -> (230, 63.9297) projected
  line L30 (225, 68.9297) -> (230, 68.9297) projected
  line L31 (225, 68.9297) -> (225, 75) projected
  line L32 (225, 75) -> (-225, 75) projected
  line L33 (-225, 75) -> (-225, 68.9297) projected
  line L34 (-225, 68.9297) -> (-230, 68.9297) projected
  line L35 (-230, 68.9297) -> (-230, 63.9297) projected
  line L36 (-230, 63.9297) -> (-225, 63.9297) projected
  line L37 (-225, 63.9297) -> (-225, 57) projected
  line L38 (-225, 57) -> (-218.8, 57) projected
  line L39 (-218.8, 57) -> (-218.8, 58.3) projected
  line L40 (-218.8, 58.3) -> (-216, 58.3) projected
  line L41 (-216, 58.3) -> (-216, 57) projected
  line L42 (-216, 57) -> (-210, 57) projected
  line L43 (-210, 57) -> (-210, 53.65) projected
  line L44 (-210, 53.65) -> (-216, 53.65) projected
  line L45 (-216, 53.65) -> (-216, 52.35) projected
  line L46 (-216, 52.35) -> (-218.8, 52.35) projected
  line L47 (-218.8, 52.35) -> (-218.8, 53.65) projected
  line L48 (-218.8, 53.65) -> (-225, 53.65) projected
  line L49 (-225, 53.65) -> (-225, 39.3833) projected
  line L50 (-225, 39.3833) -> (-230, 39.3833) projected
  line L51 (-230, 39.3833) -> (-230, 34.3833) projected
  line L52 (-230, 34.3833) -> (-225, 34.3833) projected
  line L53 (-225, 34.3833) -> (-225, 20.1167) projected
  line L54 (-225, 20.1167) -> (-218.8, 20.1167) projected
  line L55 (-218.8, 20.1167) -> (-218.8, 21.4167) projected
  line L56 (-218.8, 21.4167) -> (-216, 21.4167) projected
  line L57 (-216, 21.4167) -> (-216, 20.1167) projected
  line L58 (-216, 20.1167) -> (-210, 20.1167) projected
  line L59 (-210, 20.1167) -> (-210, 16.7667) projected
  line L60 (-210, 16.7667) -> (-216, 16.7667) projected
  line L61 (-216, 16.7667) -> (-216, 15.4667) projected
  line L62 (-216, 15.4667) -> (-218.8, 15.4667) projected
  line L63 (-218.8, 15.4667) -> (-218.8, 16.7667) projected
  line L64 (-218.8, 16.7667) -> (-225, 16.7667) projected
  line L65 (-225, 16.7667) -> (-225, 2.5) projected
  line L66 (-225, 2.5) -> (-230, 2.5) projected
  line L67 (-230, 2.5) -> (-230, -2.5) projected
  line L68 (-230, -2.5) -> (-225, -2.5) projected
  line L69 (-225, -2.5) -> (-225, -16.7667) projected
  line L70 (-225, -16.7667) -> (-218.8, -16.7667) projected
  line L71 (-218.8, -16.7667) -> (-218.8, -15.4667) projected
  line L72 (-218.8, -15.4667) -> (-216, -15.4667) projected
  line L73 (-216, -15.4667) -> (-216, -16.7667) projected
  line L74 (-216, -16.7667) -> (-210, -16.7667) projected
  line L75 (-210, -16.7667) -> (-210, -20.1167) projected
  line L76 (-210, -20.1167) -> (-216, -20.1167) projected
  line L77 (-216, -20.1167) -> (-216, -21.4167) projected
  line L78 (-216, -21.4167) -> (-218.8, -21.4167) projected
  line L79 (-218.8, -21.4167) -> (-218.8, -20.1167) projected
  line L80 (-218.8, -20.1167) -> (-225, -20.1167) projected
  line L81 (-225, -20.1167) -> (-225, -34.3833) projected
  line L82 (-225, -34.3833) -> (-230, -34.3833) projected
  line L83 (-230, -34.3833) -> (-230, -39.3833) projected
  line L84 (-230, -39.3833) -> (-225, -39.3833) projected
  line L85 (-225, -39.3833) -> (-225, -53.65) projected
  line L86 (-225, -53.65) -> (-218.8, -53.65) projected
  line L87 (-218.8, -53.65) -> (-218.8, -52.35) projected
  line L88 (-218.8, -52.35) -> (-216, -52.35) projected
  line L89 (-216, -52.35) -> (-216, -53.65) projected
  line L90 (-216, -53.65) -> (-210, -53.65) projected
  line L91 (-210, -53.65) -> (-210, -57) projected
  line L92 (-210, -57) -> (-216, -57) projected
  line L93 (-216, -57) -> (-216, -58.3) projected
  line L94 (-216, -58.3) -> (-218.8, -58.3) projected
  line L95 (-218.8, -58.3) -> (-218.8, -57) projected
  line L96 (-218.8, -57) -> (-225, -57) projected
  line L97 (-225, -57) -> (-225, -63.5) projected
  line L98 (-225, -63.5) -> (-230, -63.5) projected
  line L99 (-230, -63.5) -> (-230, -68.5) projected
  line L100 (-230, -68.5) -> (-225, -68.5) projected
  line L101 (-225, -68.5) -> (-225, -75) projected
  line L102 (-225, -75) -> (225, -75) projected
  line L103 (225, -75) -> (225, -68.5) projected
  line L104 (230, -68.5) -> (225, -68.5) projected
  line L105 (230, -63.5) -> (230, -68.5) projected
  line L106 (225, -63.5) -> (230, -63.5) projected
  line L107 (225, -63.5) -> (225, -57) projected
  line L108 (225, -57) -> (218.8, -57) projected
  line L109 (218.8, -57) -> (218.8, -58.3) projected
  line L110 (218.8, -58.3) -> (216, -58.3) projected
  line L111 (216, -58.3) -> (216, -57) projected
  line L112 (216, -57) -> (210, -57) projected
  line L113 (210, -57) -> (210, -53.65) projected
  line L114 (210, -53.65) -> (216, -53.65) projected
  line L115 (216, -53.65) -> (216, -52.35) projected
  line L116 (216, -52.35) -> (218.8, -52.35) projected
  line L117 (218.8, -52.35) -> (218.8, -53.65) projected
  line L118 (218.8, -53.65) -> (225, -53.65) projected
  line L119 (225, -53.65) -> (225, -39.3833) projected
  line L120 (230, -39.3833) -> (225, -39.3833) projected
  line L121 (230, -34.3833) -> (230, -39.3833) projected
  line L122 (225, -34.3833) -> (230, -34.3833) projected
  line L123 (225, -34.3833) -> (225, -20.1167) projected
  line L124 (225, -20.1167) -> (218.8, -20.1167) projected
  line L125 (218.8, -20.1167) -> (218.8, -21.4167) projected
  line L126 (218.8, -21.4167) -> (216, -21.4167) projected
  line L127 (216, -21.4167) -> (216, -20.1167) projected
  line L128 (216, -20.1167) -> (210, -20.1167) projected
  line L129 (210, -20.1167) -> (210, -16.7667) projected
  line L130 (210, -16.7667) -> (216, -16.7667) projected
  line L131 (216, -16.7667) -> (216, -15.4667) projected
  line L132 (216, -15.4667) -> (218.8, -15.4667) projected
  line L133 (218.8, -15.4667) -> (218.8, -16.7667) projected
  line L134 (218.8, -16.7667) -> (225, -16.7667) projected
  line L135 (225, -16.7667) -> (225, -2.5) projected
  line L136 (230, -2.5) -> (225, -2.5) projected
  line L137 (230, 2.5) -> (230, -2.5) projected
  line L138 (225, 2.5) -> (230, 2.5) projected
  line L139 (225, 2.5) -> (225, 16.7667) projected
  line L140 (-185, -75) -> (-185, -79)
  line L141 (-185, -79) -> (-155, -79)
  line L142 (-155, -79) -> (-155, -75)
  line L143 (-100, -75) -> (-100, -79)
  line L144 (-100, -79) -> (-70, -79)
  line L145 (-70, -79) -> (-70, -75)
  line L146 (-70, -75) -> (-15, -75)
  line L147 (-15, -75) -> (-15, -79)
  line L148 (-15, -79) -> (15, -79)
  line L149 (15, -79) -> (15, -75)
  line L150 (70, -75) -> (70, -79)
  line L151 (70, -79) -> (100, -79)
  line L152 (100, -79) -> (100, -75)
  line L153 (155, -75) -> (155, -79)
  line L154 (155, -79) -> (185, -79)
  line L155 (185, -79) -> (185, -75)
  line L156 (-185, -75) -> (-155, -75)
  line L157 (-100, -75) -> (-70, -75)
  line L158 (-15, -75) -> (15, -75)
  line L159 (70, -75) -> (100, -75)
  line L160 (155, -75) -> (185, -75)
  constraints: 42 end point, 5 collinear
extrude "Extrusión10" add sketch "Boceto9" against normal blind 6 contours L155 L154 L153 L102 | L152 L151 L150 L102 | L149 L148 L147 L102 | L145 L144 L143 L102 | L142 L141 L140 L102
sketch "Boceto10" plane through (0, 0, 6) normal (0, 0, 1) x (1, 0, 0)
  line L0 (-93.6885, -17.2514) -> (112.2669, -17.2514) construction
  line L1 (112.2669, -17.2514) -> (112.2669, -58.124) construction
  line L2 (112.2669, -58.124) -> (-93.6885, -58.124) construction
  line L3 (-93.6885, -58.124) -> (-93.6885, -17.2514) construction
  point P0 (0, 0)
  constraints: 2 other
extrude "Extrusión11" cut sketch "Boceto6" against normal blind 10 contours A6 | A9 | A10 | A11
extrude "Extrusión12" cut sketch "Boceto6" against normal blind 10 contours A12 | A13 | A14 | A15
extrude "Extrusión13" cut sketch "Boceto7" against normal blind 10 contours A4 | A6 | A8 | A9 | A10 | A11 | A12 | A13
sketch "Boceto12" plane through (0, 0, 6) normal (0, 0, 1) x (1, 0, 0)
  point P0 (0, 0)
sketch "Boceto13" plane through (0, 0, 6) normal (0, 0, 1) x (1, 0, 0)
  circle A0 centre (126, -15) radius 1.5 projected
  circle A1 centre (-60, 15) radius 1.5 projected
  circle A2 centre (-120, 15) radius 1.5 projected
  circle A3 centre (-90, 45) radius 1.5 projected
  circle A4 centre (126, 45) radius 1.5 projected
  circle A5 centre (-90, -15) radius 1.5 projected
  circle A6 centre (96, 15) radius 1.5 projected
  circle A7 centre (156, 15) radius 1.5 projected
  circle A8 centre (-180, -8) radius 1.5 projected
  circle A9 centre (-180, 38) radius 1.5 projected
  circle A10 centre (-203, 15) radius 1.5 projected
  circle A11 centre (-157, 15) radius 1.5 projected
  circle A12 centre (18, -8) radius 1.5 projected
  circle A13 centre (18, 38) radius 1.5 projected
  circle A14 centre (-5, 15) radius 1.5 projected
  circle A15 centre (41, 15) radius 1.5 projected
  circle A16 centre (18, 15) radius 19 projected
  circle A17 centre (126, 15) radius 21.5 projected
  circle A18 centre (-90, 15) radius 21.5 projected
  circle A19 centre (-180, 15) radius 19 projected
  line L0 (225, 16.7667) -> (218.8, 16.7667) projected
  line L1 (218.8, 16.7667) -> (218.8, 15.4667) projected
  line L2 (218.8, 15.4667) -> (216, 15.4667) projected
  line L3 (216, 15.4667) -> (216, 16.7667) projected
  line L4 (216, 16.7667) -> (210, 16.7667) projected
  line L5 (210, 16.7667) -> (210, 20.1167) projected
  line L6 (210, 20.1167) -> (216, 20.1167) projected
  line L7 (216, 20.1167) -> (216, 21.4167) projected
  line L8 (216, 21.4167) -> (218.8, 21.4167) projected
  line L9 (218.8, 21.4167) -> (218.8, 20.1167) projected
  line L10 (218.8, 20.1167) -> (225, 20.1167) projected
  line L11 (225, 20.1167) -> (225, 34.3833) projected
  line L12 (230, 34.3833) -> (225, 34.3833) projected
  line L13 (230, 39.3833) -> (230, 34.3833) projected
  line L14 (225, 39.3833) -> (230, 39.3833) projected
  line L15 (225, 39.3833) -> (225, 53.65) projected
  line L16 (225, 53.65) -> (218.8, 53.65) projected
  line L17 (218.8, 53.65) -> (218.8, 52.35) projected
  line L18 (218.8, 52.35) -> (216, 52.35) projected
  line L19 (216, 52.35) -> (216, 53.65) projected
  line L20 (216, 53.65) -> (210, 53.65) projected
  line L21 (210, 53.65) -> (210, 57) projected
  line L22 (210, 57) -> (216, 57) projected
  line L23 (216, 57) -> (216, 58.3) projected
  line L24 (216, 58.3) -> (218.8, 58.3) projected
  line L25 (218.8, 58.3) -> (218.8, 57) projected
  line L26 (218.8, 57) -> (225, 57) projected
  line L27 (225, 57) -> (225, 63.9297) projected
  line L28 (230, 63.9297) -> (225, 63.9297) projected
  line L29 (230, 68.9297) -> (230, 63.9297) projected
  line L30 (225, 68.9297) -> (230, 68.9297) projected
  line L31 (225, 68.9297) -> (225, 75) projected
  line L32 (225, 75) -> (-225, 75) projected
  line L33 (-225, 75) -> (-225, 68.9297) projected
  line L34 (-225, 68.9297) -> (-230, 68.9297) projected
  line L35 (-230, 68.9297) -> (-230, 63.9297) projected
  line L36 (-230, 63.9297) -> (-225, 63.9297) projected
  line L37 (-225, 63.9297) -> (-225, 57) projected
  line L38 (-225, 57) -> (-218.8, 57) projected
  line L39 (-218.8, 57) -> (-218.8, 58.3) projected
  line L40 (-218.8, 58.3) -> (-216, 58.3) projected
  line L41 (-216, 58.3) -> (-216, 57) projected
  line L42 (-216, 57) -> (-210, 57) projected
  line L43 (-210, 57) -> (-210, 53.65) projected
  line L44 (-210, 53.65) -> (-216, 53.65) projected
  line L45 (-216, 53.65) -> (-216, 52.35) projected
  line L46 (-216, 52.35) -> (-218.8, 52.35) projected
  line L47 (-218.8, 52.35) -> (-218.8, 53.65) projected
  line L48 (-218.8, 53.65) -> (-225, 53.65) projected
  line L49 (-225, 53.65) -> (-225, 39.3833) projected
  line L50 (-225, 39.3833) -> (-230, 39.3833) projected
  line L51 (-230, 39.3833) -> (-230, 34.3833) projected
  line L52 (-230, 34.3833) -> (-225, 34.3833) projected
  line L53 (-225, 34.3833) -> (-225, 20.1167) projected
  line L54 (-225, 20.1167) -> (-218.8, 20.1167) projected
  line L55 (-218.8, 20.1167) -> (-218.8, 21.4167) projected
  line L56 (-218.8, 21.4167) -> (-216, 21.4167) projected
  line L57 (-216, 21.4167) -> (-216, 20.1167) projected
  line L58 (-216, 20.1167) -> (-210, 20.1167) projected
  line L59 (-210, 20.1167) -> (-210, 16.7667) projected
  line L60 (-210, 16.7667) -> (-216, 16.7667) projected
  line L61 (-216, 16.7667) -> (-216, 15.4667) projected
  line L62 (-216, 15.4667) -> (-218.8, 15.4667) projected
  line L63 (-218.8, 15.4667) -> (-218.8, 16.7667) projected
  line L64 (-218.8, 16.7667) -> (-225, 16.7667) projected
  line L65 (-225, 16.7667) -> (-225, 2.5) projected
  line L66 (-225, 2.5) -> (-230, 2.5) projected
  line L67 (-230, 2.5) -> (-230, -2.5) projected
  line L68 (-230, -2.5) -> (-225, -2.5) projected
  line L69 (-225, -2.5) -> (-225, -16.7667) projected
  line L70 (-225, -16.7667) -> (-218.8, -16.7667) projected
  line L71 (-218.8, -16.7667) -> (-218.8, -15.4667) projected
  line L72 (-218.8, -15.4667) -> (-216, -15.4667) projected
  line L73 (-216, -15.4667) -> (-216, -16.7667) projected
  line L74 (-216, -16.7667) -> (-210, -16.7667) projected
  line L75 (-210, -16.7667) -> (-210, -20.1167) projected
  line L76 (-210, -20.1167) -> (-216, -20.1167) projected
  line L77 (-216, -20.1167) -> (-216, -21.4167) projected
  line L78 (-216, -21.4167) -> (-218.8, -21.4167) projected
  line L79 (-218.8, -21.4167) -> (-218.8, -20.1167) projected
  line L80 (-218.8, -20.1167) -> (-225, -20.1167) projected
  line L81 (-225, -20.1167) -> (-225, -34.3833) projected
  line L82 (-225, -34.3833) -> (-230, -34.3833) projected
  line L83 (-230, -34.3833) -> (-230, -39.3833) projected
  line L84 (-230, -39.3833) -> (-225, -39.3833) projected
  line L85 (-225, -39.3833) -> (-225, -53.65) projected
  line L86 (-225, -53.65) -> (-218.8, -53.65) projected
  line L87 (-218.8, -53.65) -> (-218.8, -52.35) projected
  line L88 (-218.8, -52.35) -> (-216, -52.35) projected
  line L89 (-216, -52.35) -> (-216, -53.65) projected
  line L90 (-216, -53.65) -> (-210, -53.65) projected
  line L91 (-210, -53.65) -> (-210, -57) projected
  line L92 (-210, -57) -> (-216, -57) projected
  line L93 (-216, -57) -> (-216, -58.3) projected
  line L94 (-216, -58.3) -> (-218.8, -58.3) projected
  line L95 (-218.8, -58.3) -> (-218.8, -57) projected
  line L96 (-218.8, -57) -> (-225, -57) projected
  line L97 (-225, -57) -> (-225, -63.5) projected
  line L98 (-225, -63.5) -> (-230, -63.5) projected
  line L99 (-230, -63.5) -> (-230, -68.5) projected
  line L100 (-230, -68.5) -> (-225, -68.5) projected
  line L101 (-225, -68.5) -> (-225, -75) projected
  line L102 (-225, -75) -> (-185, -75) projected
  line L103 (-185, -75) -> (-185, -79) projected
  line L104 (-185, -79) -> (-155, -79) projected
  line L105 (-155, -79) -> (-155, -75) projected
  line L106 (-155, -75) -> (-100, -75) projected
  line L107 (-100, -75) -> (-100, -79) projected
  line L108 (-100, -79) -> (-70, -79) projected
  line L109 (-70, -79) -> (-70, -75) projected
  line L110 (-70, -75) -> (-15, -75) projected
  line L111 (-15, -75) -> (-15, -79) projected
  line L112 (-15, -79) -> (15, -79) projected
  line L113 (15, -79) -> (15, -75) projected
  line L114 (15, -75) -> (70, -75) projected
  line L115 (70, -75) -> (70, -79) projected
  line L116 (70, -79) -> (100, -79) projected
  line L117 (100, -79) -> (100, -75) projected
  line L118 (100, -75) -> (155, -75) projected
  line L119 (155, -79) -> (155, -75) projected
  line L120 (185, -79) -> (155, -79) projected
  line L121 (185, -75) -> (185, -79) projected
  line L122 (185, -75) -> (225, -75) projected
  line L123 (225, -75) -> (225, -68.5) projected
  line L124 (230, -68.5) -> (225, -68.5) projected
  line L125 (230, -63.5) -> (230, -68.5) projected
  line L126 (225, -63.5) -> (230, -63.5) projected
  line L127 (225, -63.5) -> (225, -57) projected
  line L128 (225, -57) -> (218.8, -57) projected
  line L129 (218.8, -57) -> (218.8, -58.3) projected
  line L130 (218.8, -58.3) -> (216, -58.3) projected
  line L131 (216, -58.3) -> (216, -57) projected
  line L132 (216, -57) -> (210, -57) projected
  line L133 (210, -57) -> (210, -53.65) projected
  line L134 (210, -53.65) -> (216, -53.65) projected
  line L135 (216, -53.65) -> (216, -52.35) projected
  line L136 (216, -52.35) -> (218.8, -52.35) projected
  line L137 (218.8, -52.35) -> (218.8, -53.65) projected
  line L138 (218.8, -53.65) -> (225, -53.65) projected
  line L139 (225, -53.65) -> (225, -39.3833) projected
  line L140 (230, -39.3833) -> (225, -39.3833) projected
  line L141 (230, -34.3833) -> (230, -39.3833) projected
  line L142 (225, -34.3833) -> (230, -34.3833) projected
  line L143 (225, -34.3833) -> (225, -20.1167) projected
  line L144 (225, -20.1167) -> (218.8, -20.1167) projected
  line L145 (218.8, -20.1167) -> (218.8, -21.4167) projected
  line L146 (218.8, -21.4167) -> (216, -21.4167) projected
  line L147 (216, -21.4167) -> (216, -20.1167) projected
  line L148 (216, -20.1167) -> (210, -20.1167) projected
  line L149 (210, -20.1167) -> (210, -16.7667) projected
  line L150 (210, -16.7667) -> (216, -16.7667) projected
  line L151 (216, -16.7667) -> (216, -15.4667) projected
  line L152 (216, -15.4667) -> (218.8, -15.4667) projected
  line L153 (218.8, -15.4667) -> (218.8, -16.7667) projected
  line L154 (218.8, -16.7667) -> (225, -16.7667) projected
  line L155 (225, -16.7667) -> (225, -2.5) projected
  line L156 (230, -2.5) -> (225, -2.5) projected
  line L157 (230, 2.5) -> (230, -2.5) projected
  line L158 (225, 2.5) -> (230, 2.5) projected
  line L159 (225, 2.5) -> (225, 16.7667) projected
  circle A20 centre (-90, 15) radius 26.5
  circle A21 centre (126, 15) radius 26.5
  point P0 (0, 0)
  dimension "d177" = 53
  dimension "d178" = 53
  constraints: 2 centre point, 2 coincident
  measures "d177" diameter of A20
  measures "d178" diameter of A21
extrude "Extrusión14" cut sketch "Boceto13" against normal blind 10 contours A20 | A21
sketch "Boceto14" plane through (230, -68.5, 6) normal (1, 0, 0) x (0, 0, -1)
  line L0 (0, 5) -> (0, 0) projected
  line L1 (0, 0) -> (6, 0) projected
  line L2 (6, 0) -> (6, 5) projected
  line L3 (0, 5) -> (6, 5) projected
  line L4 (0, 34.1167) -> (0, 29.1167) projected
  line L5 (0, 29.1167) -> (6, 29.1167) projected
  line L6 (6, 29.1167) -> (6, 34.1167) projected
  line L7 (0, 34.1167) -> (6, 34.1167) projected
  line L8 (0, 71) -> (0, 66) projected
  line L9 (0, 66) -> (6, 66) projected
  line L10 (6, 66) -> (6, 71) projected
  line L11 (0, 71) -> (6, 71) projected
  line L12 (0, 107.8833) -> (0, 102.8833) projected
  line L13 (0, 102.8833) -> (6, 102.8833) projected
  line L14 (6, 102.8833) -> (6, 107.8833) projected
  line L15 (0, 107.8833) -> (6, 107.8833) projected
  line L16 (0, 137.4297) -> (0, 132.4297) projected
  line L17 (0, 132.4297) -> (6, 132.4297) projected
  line L18 (6, 132.4297) -> (6, 137.4297) projected
  line L19 (0, 137.4297) -> (6, 137.4297) projected
  point P0 (6, 68.5)
extrude "Extrusión15" add sketch "Boceto14" along normal blind 1
mirror "Simetría3" about plane through (0, 0, 0) normal (1, 0, 0) of "Extrusión15"
fillet "Empalme1" radius 2 4 edges at (-199, 15, 6) (-116.5, 15, 6) (-1, 15, 6) (99.5, 15, 6)
equation "\"d73\" = d72"
